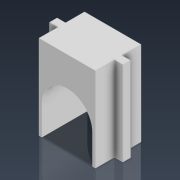
# Autodesk Inventor part: Slider-1
Saved by Autodesk Inventor 2021.1 (Build 251245010, 245A)
## iProperties
Created: 2020-12-20
Part Number: Slider-1
Material: 一般
Document SubType Name: Modeling
Designer: User
Density: 1 g/cm^3
Appearance: 預設
Author: User
Autodesk Inventor part; units mm, degrees
ref_plane "YZ Plane" through (0, 0, 0) normal (1, 0, 0) x (0, 1, 0)
ref_plane "XZ Plane" through (0, 0, 0) normal (0, 1, 0) x (-1, 0, 0)
ref_plane "XY Plane" through (0, 0, 0) normal (0, 0, 1) x (1, 0, 0)
sketch "草圖1" plane through (0, 0, 0) normal (0, 1, 0) x (-1, 0, 0)
  line L0 (-33.5, 27) -> (33.5, 27)
  line L1 (33.5, 27) -> (33.5, -27)
  line L2 (33.5, -27) -> (-33.5, -27)
  line L3 (-33.5, -27) -> (-33.5, 27)
  line L4 (-33.5, 27) -> (33.5, -27) construction
  line L5 (33.5, 27) -> (-33.5, -27) construction
  line L6 (43.5, -4.5) -> (33.5, -4.5)
  line L7 (33.5, -4.5) -> (33.5, 4.5)
  line L8 (33.5, 4.5) -> (43.5, 4.5)
  line L9 (43.5, 4.5) -> (43.5, -4.5)
  line L10 (-33.5, -4.5) -> (-43.5, -4.5)
  line L11 (-43.5, -4.5) -> (-43.5, 4.5)
  line L12 (-43.5, 4.5) -> (-33.5, 4.5)
  line L13 (-33.5, 4.5) -> (-33.5, -4.5)
  point P0 (0, 0)
  point P1 (33.5, 0)
  point P2 (-33.5, 0)
  point P3 (-33.5, 4.5)
  point P4 (-33.5, -4.5)
  dimension "d0" = 67
  dimension "d1" = 54
  dimension "d2" = 9
  dimension "d3" = 10
  constraints: 28 end point, 6 midpoint, 6 parallel, 3 horizontal, 3 perpendicular, 2 equal length
  measures "d0" distance of L0.start L0.end
  measures "d1" distance of L2.end L0.start
  measures "d2" distance of L8.end L6.start
  measures "d3" distance of L6.start L6.end
extrude "擠出1" add sketch "草圖1" along normal blind 100
sketch "草圖2" plane through (-33.5, 0, 27) normal (0, 0, 1) x (1, 0, 0)
  circle A0 centre (33.5, 33) radius 30
  line L0 (0, 0) -> (67, 0) projected
  line L1 (3.5, 33) -> (63.5, 33)
  line L2 (63.5, 33) -> (63.5, -12.4903)
  line L3 (63.5, -12.4903) -> (3.5, -12.4903)
  line L4 (3.5, -12.4903) -> (3.5, 33)
  point P0 (33.5, 0)
  point P1 (33.5, 0)
  point P2 (63.5, 33)
  dimension "d6" = 33
  dimension "d7" = 60
  constraints: 8 end point, 2 midpoint, 2 parallel, 2 tangent, 1 centre point, 1 coincident, 1 horizontal, 1 perpendicular, 1 vertical alignment
  measures "d6" distance from line of L0 A0.centre
  measures "d7" diameter of A0
extrude "擠出2" cut sketch "草圖2" against normal through all
sketch "草圖3" plane through (33.5, 100, -27) normal (0, 0, -1) x (-1, 0, 0)
  line L0 (3.5, -100) -> (3.5, -67) projected
  arc A0 (63.5, -67) -> (3.5, -67) centre (33.5, -67) ccw projected
  line L1 (63.5, -67) -> (63.5, -100) projected
  line L2 (63.5, -100) -> (67, -100) projected
  line L3 (67, -100) -> (67, 0) projected
  line L4 (0, 0) -> (67, 0) projected
  line L5 (0, -100) -> (0, 0) projected
  line L6 (0, -100) -> (3.5, -100) projected
  line L7 (63.5, -67) -> (63.5, -100) projected
  line L8 (63.5, -100) -> (3.5, -100)
  point P0 (33.5, -100)
  constraints: 2 end point, 1 perpendicular
sketch "草圖4" plane through (-33.5, 100, 27) normal (0, 0, 1) x (1, 0, 0)
  circle A0 centre (33.5, -65) radius 30
  arc A1 (63.5, -67) -> (3.5, -67) centre (33.5, -67) ccw construction
  line L0 (63.5, -100) -> (3.5, -100)
  line L1 (3.5, -100) -> (3.5, -65)
  line L2 (3.5, -65) -> (63.5, -65)
  line L3 (63.5, -65) -> (63.5, -100)
  point P0 (33.5, -100)
  dimension "d10" = 60
  dimension "d11" = 2
  constraints: 8 end point, 2 coincident, 2 parallel, 1 centre point, 1 horizontal, 1 midpoint, 1 perpendicular, 1 tangent, 1 vertical alignment
  measures "d10" diameter of A0
  measures "d11" distance of A1.centre A0.centre
loft "斷面混成1" cut profiles "草圖3", "草圖4" contours L0 A0 L1 L8 / all
